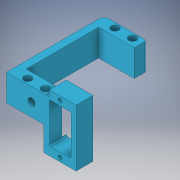
# Autodesk Inventor part: 000.701 - Опора
Saved by Autodesk Inventor 2019 (Build 230136000, 136)
## iProperties
Created: 2020-02-29
Part Number: 000.701 - Опора
Material: Пластик АБС
Document SubType Name: Modeling
Designer: Петров Иван
Density: 1.06 g/cm^3
Appearance: Бирюзовый
Author: Петров Иван
Autodesk Inventor part; units mm, degrees
ref_plane "YZ Plane" through (0, 0, 0) normal (1, 0, 0) x (0, 1, 0)
ref_plane "XZ Plane" through (0, 0, 0) normal (0, 1, 0) x (-1, 0, 0)
ref_plane "XY Plane" through (0, 0, 0) normal (0, 0, 1) x (1, 0, 0)
sketch "Эскиз1" plane through (0, 0, 0) normal (0, 1, 0) x (-1, 0, 0)
  line L0 (-3.75, -37.7) -> (-0.5, -37.7)
  line L1 (-0.5, -37.7) -> (-0.5, -30.7)
  line L2 (-0.5, -30.7) -> (-10, -30.7)
  line L3 (-10, -30.7) -> (-10, -36.7)
  arc A0 (-10, -36.7) -> (-9, -37.7) centre (-9, -36.7) ccw
  line L4 (-9, -37.7) -> (-6.15, -37.7)
  line L5 (-6.15, -37.7) -> (-6.15, -36.634)
  arc A1 (-3.75, -36.634) -> (-6.15, -36.634) centre (-4.95, -34.85) ccw
  line L6 (-3.75, -36.634) -> (-3.75, -37.7)
  line L7 (0.5, -37.7) -> (0.5, -30.7)
  line L8 (0.5, -37.7) -> (3.75, -37.7)
  line L9 (3.75, -37.7) -> (3.75, -36.634)
  arc A2 (6.15, -36.634) -> (3.75, -36.634) centre (4.95, -34.85) ccw
  line L10 (6.15, -36.634) -> (6.15, -37.7)
  line L11 (6.15, -37.7) -> (9, -37.7)
  arc A3 (9, -37.7) -> (10, -36.7) centre (9, -36.7) ccw
  line L12 (10, -36.7) -> (10, -30.7)
  line L13 (10, -30.7) -> (0.5, -30.7)
  line L14 (0.5, 10) -> (0.5, 17)
  line L15 (10, 10) -> (0.5, 10)
  line L16 (10, 16) -> (10, 10)
  arc A4 (10, 16) -> (9, 17) centre (9, 16) ccw
  line L17 (6.15, 17) -> (9, 17)
  line L18 (6.15, 15.934) -> (6.15, 17)
  arc A5 (3.75, 15.934) -> (6.15, 15.934) centre (4.95, 14.15) ccw
  line L19 (3.75, 17) -> (3.75, 15.934)
  line L20 (0.5, 17) -> (3.75, 17)
  line L21 (-0.5, 10) -> (-10, 10)
  line L22 (-0.5, 10) -> (-0.5, 17)
  line L23 (-3.75, 17) -> (-0.5, 17)
  line L24 (-3.75, 15.934) -> (-3.75, 17)
  arc A6 (-6.15, 15.934) -> (-3.75, 15.934) centre (-4.95, 14.15) ccw
  line L25 (-6.15, 17) -> (-6.15, 15.934)
  line L26 (-9, 17) -> (-6.15, 17)
  arc A7 (-9, 17) -> (-10, 16) centre (-9, 16) ccw
  line L27 (-10, 10) -> (-10, 16)
  line L28 (-10, -30.7) -> (-10, 0)
  line L29 (-10, 0) -> (-10, 10)
  line L30 (10, 0) -> (10, 10)
  line L31 (10, -30.7) -> (10, 0)
  circle A8 centre (0, 0) radius 6.5
  circle A9 centre (0, 0) radius 5.4
  circle A10 centre (0, 0) radius 3.4957
  circle A11 centre (0, 0) radius 3.4957
  circle A12 centre (-4.95, -34.85) radius 2.15
  circle A13 centre (4.95, -34.85) radius 2.15
  arc A14 (-6.15, 15.934) -> (-3.75, 15.934) centre (-4.95, 14.15) ccw
  circle A15 centre (-4.95, 14.15) radius 2.15
  circle A16 centre (4.95, 14.15) radius 2.15
  line L32 (-3.75, -37.7) -> (-0.5, -37.7)
  line L33 (-6.15, -37.7) -> (-3.75, -37.7)
  line L34 (-3.75, -37.7) -> (3.75, -37.7)
  line L35 (3.75, -37.7) -> (6.15, -37.7)
  line L36 (-6.15, 17) -> (-3.75, 17)
  line L37 (3.75, 17) -> (3.75, 15.934)
  line L38 (3.75, 17) -> (6.15, 17)
  line L39 (0.5, 17) -> (-0.5, 17)
  line L40 (0.5, 10) -> (-0.5, 10)
  line L41 (0.5, -30.7) -> (-0.5, -30.7)
  point P0 (10, -10.35)
  constraints: 84 end point, 18 point on circle, 15 centre point, 4 coincident, 2 concentric, 2 horizontal, 1 collinear, 1 parallel, 1 perpendicular, 6 other
extrude "Выдавливание1" add sketch "Эскиз1" along normal blind 15 contours L6 A1 L5 L4 A0 L3 L2 L1 L0 | L33 L5 A12 L6 | L1 L41 L7 L34 | L7 L13 L12 A3 L11 L10 A2 L9 L8 | L9 A13 L10 L35 | L27 A7 L26 L25 A6 L24 L23 L22 L21 | L22 L39 L14 L40 | L15 L14 L20 L19 A5 L18 L17 A4 L16 | L24 A15 L25 L36 | L38 L18 A16 L19
sketch "Эскиз2" plane through (-10, 0, -36.7) normal (-1, 0, 0) x (0, 0, 1)
  line L0 (6, 15) -> (0, 15) projected
  line L1 (46.7, 0) -> (52.7, 0) projected
  line L2 (0, 15) -> (52.7, 15)
  line L3 (52.7, 15) -> (52.7, 0)
  line L4 (52.7, 0) -> (0, 0)
  line L5 (0, 0) -> (0, 15)
  point P0 (36.7, 0)
  constraints: 8 end point, 2 parallel, 1 horizontal, 1 perpendicular
extrude "Выдавливание2" add sketch "Эскиз2" along normal blind 4
move faces "Перенос2" translate (0, 0, 1) faces at (-11.3333, 10, 16)
move faces "Перенос3" translate (0, 0, -1) faces at (-11.3333, 5, -36.7)
chamfer "Фаска8" distance 2 angle 45 1 edges at (-14, 7.5, -37.7)
sketch "Эскиз16" plane through (0, 15, 0) normal (0, 1, 0) x (1, 0, 0)
  line L0 (10, -16) -> (10, -10) projected
  arc A0 (9, -17) -> (10, -16) centre (9, -16) ccw projected
  line L1 (10, -16) -> (9, -16)
  line L2 (9, -16) -> (9, -17)
  line L3 (9, -17) -> (10, -17)
  line L4 (10, -17) -> (10, -16)
  point P0 (0, 0)
  constraints: 8 end point, 2 parallel, 1 horizontal, 1 perpendicular
extrude "Выдавливание16" add sketch "Эскиз16" against normal up to surface (15 mm away)
sketch "Эскиз20" plane through (-14, 15, 17) normal (0, 0, 1) x (1, 0, 0)
  line L0 (14, -15) -> (14, 0)
  line L1 (4, 0) -> (24, 0) projected
  circle A0 centre (14, -7.5) radius 2
  dimension "d102" = 4
  constraints: 2 end point, 2 midpoint, 1 centre point
  measures "d102" diameter of A0
extrude "Выдавливание20" cut sketch "Эскиз20" against normal blind 12.5
sketch "Эскиз21" plane through (10, 0, 10) normal (0, 0, -1) x (-1, 0, 0)
  circle A0 centre (10, 7.5) radius 2 projected
  circle A1 centre (10, 7.5) radius 4
  point P0 (10, 0)
  dimension "d105" = 8
  constraints: 1 centre point, 1 coincident
  measures "d105" diameter of A1
extrude "Выдавливание21" cut sketch "Эскиз21" against normal blind 3
sketch "Эскиз22" plane through (-14, 15, 17) normal (0, 0, 1) x (1, 0, 0)
  line L0 (33, -12.98) -> (33, -13.1)
  arc A0 (27.2, -13.1) -> (33, -13.1) centre (30.1, -13.1) ccw
  line L1 (27.2, -13.1) -> (27.2, -12.98)
  arc A1 (24.1, -9.062) -> (27.2, -12.98) centre (30.1, -7.5) ccw
  line L2 (24.1, -9.062) -> (24.1, -23.05)
  arc A2 (24.1, -23.05) -> (24.85, -23.8) centre (24.85, -23.05) ccw
  line L3 (24.85, -23.8) -> (35.35, -23.8)
  arc A3 (35.35, -23.8) -> (36.1, -23.05) centre (35.35, -23.05) ccw
  line L4 (36.1, -23.05) -> (36.1, -9.062)
  arc A4 (33, -12.98) -> (36.1, -9.062) centre (30.1, -7.5) ccw
  line L5 (25, -17.4) -> (25, -22.4)
  arc A5 (25.5, -16.9) -> (25, -17.4) centre (25.5, -17.4) ccw
  line L6 (34.7, -16.9) -> (25.5, -16.9)
  arc A6 (35.2, -17.4) -> (34.7, -16.9) centre (34.7, -17.4) ccw
  line L7 (35.2, -22.4) -> (35.2, -17.4)
  arc A7 (34.7, -22.9) -> (35.2, -22.4) centre (34.7, -22.4) ccw
  line L8 (25.5, -22.9) -> (34.7, -22.9)
  arc A8 (25, -22.4) -> (25.5, -22.9) centre (25.5, -22.4) ccw
  arc A9 (30.65, -27.5026) -> (29.55, -27.5026) centre (30.1, -26.55) ccw
  line L9 (30.65, -28.7) -> (30.65, -27.5026)
  line L10 (30.65, -28.7) -> (35.35, -28.7)
  arc A10 (35.35, -28.7) -> (36.2, -27.85) centre (35.35, -27.85) ccw
  line L11 (36.2, -27.85) -> (36.2, -23.05)
  arc A11 (35.35, -23.9) -> (36.2, -23.05) centre (35.35, -23.05) ccw
  line L12 (24.85, -23.9) -> (35.35, -23.9)
  arc A12 (24, -23.05) -> (24.85, -23.9) centre (24.85, -23.05) ccw
  line L13 (24, -23.05) -> (24, -27.85)
  arc A13 (24, -27.85) -> (24.85, -28.7) centre (24.85, -27.85) ccw
  line L14 (24.85, -28.7) -> (29.55, -28.7)
  line L15 (29.55, -27.5026) -> (29.55, -28.7)
  line L16 (35.35, 3.4) -> (30.65, 3.4)
  line L17 (30.65, 2.2026) -> (30.65, 3.4)
  arc A14 (29.55, 2.2026) -> (30.65, 2.2026) centre (30.1, 1.25) ccw
  line L18 (29.55, 3.4) -> (29.55, 2.2026)
  line L19 (29.55, 3.4) -> (24.85, 3.4)
  arc A15 (24.85, 3.4) -> (24, 2.55) centre (24.85, 2.55) ccw
  line L20 (24, 2.55) -> (24, -2.25)
  arc A16 (24.85, -1.4) -> (24, -2.25) centre (24.85, -2.25) ccw
  line L21 (35.35, -1.4) -> (24.85, -1.4)
  arc A17 (36.2, -2.25) -> (35.35, -1.4) centre (35.35, -2.25) ccw
  line L22 (36.2, -2.25) -> (36.2, 2.55)
  arc A18 (36.2, 2.55) -> (35.35, 3.4) centre (35.35, 2.55) ccw
  line L23 (36.2, -2.25) -> (36.2, -5.938)
  line L24 (36.2, -9.062) -> (36.2, -7.5)
  line L25 (36.2, -7.5) -> (36.2, -5.938)
  line L26 (36.2, -9.062) -> (36.2, -23.05)
  line L27 (24, -23.05) -> (24, -9.062)
  line L28 (24, -5.938) -> (24, -2.25)
  line L29 (24, -5.938) -> (24, -7.5)
  line L30 (24, -7.5) -> (24, -9.062)
  arc A19 (36.1, -5.938) -> (31.662, -1.5) centre (30.1, -7.5) ccw
  line L31 (36.1, -5.938) -> (36.1, -2.25)
  arc A20 (36.1, -2.25) -> (35.35, -1.5) centre (35.35, -2.25) ccw
  line L32 (35.35, -1.5) -> (31.662, -1.5)
  line L33 (24.1, -2.25) -> (24.1, -5.938)
  arc A21 (28.538, -1.5) -> (24.1, -5.938) centre (30.1, -7.5) ccw
  line L34 (28.538, -1.5) -> (24.85, -1.5)
  arc A22 (24.85, -1.5) -> (24.1, -2.25) centre (24.85, -2.25) ccw
  circle A23 centre (30.1, -26.55) radius 1.1
  line L35 (30.65, -27.5026) -> (30.65, -28.7)
  line L36 (29.55, -28.7) -> (30.65, -28.7)
  circle A24 centre (30.1, 1.25) radius 1.1
  line L37 (30.65, 3.4) -> (30.65, 2.2026)
  line L38 (29.55, 3.4) -> (30.65, 3.4)
  circle A25 centre (30.1, -7.5) radius 0.8
  line L39 (24, -15) -> (24, 0) projected
  line L40 (24, -7.5) -> (30.1, -7.5)
  line L41 (24, -28.7) -> (39, -28.7)
  line L42 (39, -28.7) -> (39, 3.4)
  line L43 (39, 3.4) -> (24, 3.4)
  line L44 (24, 3.4) -> (24, -28.7)
  line L45 (24, -15) -> (4, -15) projected
  line L46 (24, -28.7) -> (21, -28.7)
  line L47 (21, -28.7) -> (21, -15)
  line L48 (21, -15) -> (24, -15)
  line L49 (24, -15) -> (24, -28.7)
  point P0 (14, -15)
  point P1 (30.1, -12.65)
  dimension "d108" = 6.1
  dimension "d109" = 15
  dimension "d112" = 3
  constraints: 96 end point, 46 point on circle, 25 centre point, 4 parallel, 3 horizontal, 2 coincident, 2 perpendicular, 1 collinear, 1 concentric, 1 midpoint, 1 point on line, 3 other
  measures "d108" distance of L40.start L40.end
  measures "d109" distance of L43.end L42.end
  measures "d112" distance of L47.end L48.end
extrude "Выдавливание22" add sketch "Эскиз22" against normal blind 7 contours A9 L15 L14 A13 L13 A12 L12 A11 L11 A10 L10 L9 | L9 L36 L15 A23 | A10 L11 L26 L24 L25 L23 L22 A18 L43 L42 L41 | L41 L44 A13 | L44 L46 L47 L45 L27 L13 | A18 L22 A17 L21 A16 L20 A15 L19 L18 A14 L17 L16 | L17 A24 L18 L38 | A15 L44 L43
sketch "Эскиз23" plane through (-10, 0, 10) normal (0, 0, -1) x (-1, 0, 0)
  line L0 (-29, 2.68) -> (-29, 2.8)
  arc A0 (-23.2, 2.8) -> (-29, 2.8) centre (-26.1, 2.8) ccw
  line L1 (-23.2, 2.8) -> (-23.2, 2.68)
  arc A1 (-20.1, -1.238) -> (-23.2, 2.68) centre (-26.1, -2.8) ccw
  line L2 (-20.1, -1.238) -> (-20.1, 12.75)
  arc A2 (-20.1, 12.75) -> (-20.85, 13.5) centre (-20.85, 12.75) ccw
  line L3 (-20.85, 13.5) -> (-31.35, 13.5)
  arc A3 (-31.35, 13.5) -> (-32.1, 12.75) centre (-31.35, 12.75) ccw
  line L4 (-32.1, 12.75) -> (-32.1, -1.238)
  arc A4 (-29, 2.68) -> (-32.1, -1.238) centre (-26.1, -2.8) ccw
  line L5 (-21, 7.1) -> (-21, 12.1)
  arc A5 (-21.5, 6.6) -> (-21, 7.1) centre (-21.5, 7.1) ccw
  line L6 (-30.7, 6.6) -> (-21.5, 6.6)
  arc A6 (-31.2, 7.1) -> (-30.7, 6.6) centre (-30.7, 7.1) ccw
  line L7 (-31.2, 12.1) -> (-31.2, 7.1)
  arc A7 (-30.7, 12.6) -> (-31.2, 12.1) centre (-30.7, 12.1) ccw
  line L8 (-21.5, 12.6) -> (-30.7, 12.6)
  arc A8 (-21, 12.1) -> (-21.5, 12.6) centre (-21.5, 12.1) ccw
  arc A9 (-26.65, 17.2026) -> (-25.55, 17.2026) centre (-26.1, 16.25) ccw
  line L9 (-26.65, 18.4) -> (-26.65, 17.2026)
  line L10 (-26.65, 18.4) -> (-31.35, 18.4)
  arc A10 (-31.35, 18.4) -> (-32.2, 17.55) centre (-31.35, 17.55) ccw
  line L11 (-32.2, 17.55) -> (-32.2, 12.75)
  arc A11 (-31.35, 13.6) -> (-32.2, 12.75) centre (-31.35, 12.75) ccw
  line L12 (-20.85, 13.6) -> (-31.35, 13.6)
  arc A12 (-20, 12.75) -> (-20.85, 13.6) centre (-20.85, 12.75) ccw
  line L13 (-20, 12.75) -> (-20, 17.55)
  arc A13 (-20, 17.55) -> (-20.85, 18.4) centre (-20.85, 17.55) ccw
  line L14 (-20.85, 18.4) -> (-25.55, 18.4)
  line L15 (-25.55, 17.2026) -> (-25.55, 18.4)
  line L16 (-31.35, -13.7) -> (-26.65, -13.7)
  line L17 (-26.65, -12.5026) -> (-26.65, -13.7)
  arc A14 (-25.55, -12.5026) -> (-26.65, -12.5026) centre (-26.1, -11.55) ccw
  line L18 (-25.55, -13.7) -> (-25.55, -12.5026)
  line L19 (-25.55, -13.7) -> (-20.85, -13.7)
  arc A15 (-20.85, -13.7) -> (-20, -12.85) centre (-20.85, -12.85) ccw
  line L20 (-20, -12.85) -> (-20, -8.05)
  arc A16 (-20.85, -8.9) -> (-20, -8.05) centre (-20.85, -8.05) ccw
  line L21 (-31.35, -8.9) -> (-20.85, -8.9)
  arc A17 (-32.2, -8.05) -> (-31.35, -8.9) centre (-31.35, -8.05) ccw
  line L22 (-32.2, -8.05) -> (-32.2, -12.85)
  arc A18 (-32.2, -12.85) -> (-31.35, -13.7) centre (-31.35, -12.85) ccw
  line L23 (-32.2, -8.05) -> (-32.2, -4.362)
  line L24 (-32.2, -1.238) -> (-32.2, -2.8)
  line L25 (-32.2, -2.8) -> (-32.2, -4.362)
  line L26 (-32.2, -1.238) -> (-32.2, 12.75)
  line L27 (-20, 12.75) -> (-20, -1.238)
  line L28 (-20, -4.362) -> (-20, -8.05)
  line L29 (-20, -4.362) -> (-20, -2.8)
  line L30 (-20, -2.8) -> (-20, -1.238)
  arc A19 (-32.1, -4.362) -> (-27.662, -8.8) centre (-26.1, -2.8) ccw
  line L31 (-32.1, -4.362) -> (-32.1, -8.05)
  arc A20 (-32.1, -8.05) -> (-31.35, -8.8) centre (-31.35, -8.05) ccw
  line L32 (-31.35, -8.8) -> (-27.662, -8.8)
  line L33 (-20.1, -8.05) -> (-20.1, -4.362)
  arc A21 (-24.538, -8.8) -> (-20.1, -4.362) centre (-26.1, -2.8) ccw
  line L34 (-24.538, -8.8) -> (-20.85, -8.8)
  arc A22 (-20.85, -8.8) -> (-20.1, -8.05) centre (-20.85, -8.05) ccw
  circle A23 centre (-26.1, 16.25) radius 1.1
  line L35 (-26.65, 17.2026) -> (-26.65, 18.4)
  line L36 (-25.55, 18.4) -> (-26.65, 18.4)
  circle A24 centre (-26.1, -11.55) radius 1.1
  line L37 (-26.65, -13.7) -> (-26.65, -12.5026)
  line L38 (-25.55, -13.7) -> (-26.65, -13.7)
  circle A25 centre (-26.1, -2.8) radius 0.8
  line L39 (-20, 4.7) -> (-20, -10.3)
  line L40 (-20, -2.8) -> (-26.1, -2.8)
  line L41 (-20, 18.4) -> (-35, 18.4)
  line L42 (-35, 18.4) -> (-35, -13.7)
  line L43 (-35, -13.7) -> (-20, -13.7)
  line L44 (-20, -13.7) -> (-20, 18.4)
  line L45 (-20, 4.7) -> (0, 4.7)
  line L46 (-20, 18.4) -> (-17, 18.4)
  line L47 (-17, 18.4) -> (-17, 4.7)
  line L48 (-17, 4.7) -> (-20, 4.7)
  line L49 (-20, 4.7) -> (-20, 18.4)
  line L50 (-35, 18.4) -> (-35, -13.7) projected
  point P0 (-10, 0)
  point P1 (-10, 4.7)
  point P2 (-26.1, 2.35)
  dimension "d122" = 6.1
  dimension "d123" = 15
  dimension "d124" = 3
  constraints: 100 end point, 46 point on circle, 25 centre point, 4 parallel, 2 coincident, 2 perpendicular, 1 collinear, 1 concentric, 1 midpoint, 1 point on line, 3 other
  measures "d122" distance of L40.start L40.end
  measures "d123" distance of L43.end L42.end
  measures "d124" distance of L47.end L48.end
extrude "Выдавливание23" add sketch "Эскиз23" along normal blind 2.5 contours A9 L15 L14 A13 L13 A12 L12 A11 L11 A10 L10 L9 | L9 L36 L15 A23 | A10 L11 L26 L24 L25 L23 L22 A18 L43 L42 L41 | L41 L44 A13 | A18 L22 A17 L21 A16 L20 A15 L19 L18 A14 L17 L16 | L17 A24 L18 L38 | A15 L44 L43
sketch "Эскиз24" plane through (-14, 0, 17) normal (0, 0, 1) x (1, 0, 0)
  circle A0 centre (14, 7.5) radius 2 projected
  circle A1 centre (14, 7.5) radius 2
  point P0 (14, 0)
  constraints: 1 centre point, 1 coincident
extrude "Выдавливание24" [suppressed]
